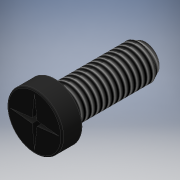
# Autodesk Inventor part: m5x12mmscrew
Saved by Autodesk Inventor 2018 (Build 220112000, 112)
## iProperties
Created: 2017-11-24
Part Number: m5x12mmscrew
Material: Generic
Document SubType Name: Modeling
Designer: g
Density: 1 g/cm^3
Appearance: Default
Author: g
Autodesk Inventor part; units mm, degrees
ref_plane "YZ Plane" through (0, 0, 0) normal (1, 0, 0) x (0, 1, 0)
ref_plane "XZ Plane" through (0, 0, 0) normal (0, 1, 0) x (-1, 0, 0)
ref_plane "XY Plane" through (0, 0, 0) normal (0, 0, 1) x (1, 0, 0)
sketch "Sketch1" plane through (0, 0, 0) normal (0, 1, 0) x (-1, 0, 0)
  circle A0 centre (0, 0) radius 2.5
  circle A1 centre (0, 0) radius 4
  dimension "d0" = 5
  dimension "d1" = 8
  constraints: 2 centre point, 2 coincident
  measures "d0" diameter of A0
  measures "d1" diameter of A1
extrude "Extrusion1" add sketch "Sketch1" along normal blind 15 contours A0
extrude "Extrusion2" add sketch "Sketch1" along normal blind 3
sketch "Sketch3" plane through (0, 0, 0) normal (0, -1, 0) x (1, 0, 0)
  line L0 (0, 0) -> (0, -0.4) construction
  circle A0 centre (0, 0) radius 4 projected
  line L1 (4, 0) -> (3.5, 0) construction
  line L2 (0, 0) -> (0, 0.4) construction
  line L3 (0.359, 0.359) -> (3.5, 0)
  line L4 (3.5, 0) -> (0.359, -0.359)
  line L5 (0.359, -0.359) -> (0, -3.5)
  line L6 (-0.359, -0.359) -> (0, -3.5)
  line L7 (-0.359, -0.359) -> (-3.5, 0)
  line L8 (-3.5, 0) -> (-0.359, 0.359)
  line L9 (-0.359, 0.359) -> (0, 3.5)
  line L10 (0, 3.5) -> (0.359, 0.359)
  dimension "d14" = 0.4
  dimension "d15" = 0.5
  dimension "d16" = 0.4
  dimension "d21" = 103.04
  dimension "d22" = 103.04
  dimension "d23" = 13.04
  dimension "d24" = 3.1615
  dimension "d25" = 3.1615
  constraints: 22 end point, 3 perpendicular, 2 horizontal, 2 vertical, 1 horizontal alignment, 1 other
  measures "d14" distance of L0.start L0.end
  measures "d15" distance of L1.start L1.end
  measures "d16" distance of L2.start L2.end
  measures "d21" angle of L8 L9
  measures "d22" angle of L3 L10
  measures "d23" angle of L10 L9
  measures "d24" distance of L8.end L9.end
  measures "d25" distance of L9.end L3.start
extrude "Extrusion3" cut sketch "Sketch3" against normal blind 2 contours L3 L4 L5 L6 L7 L8 L9 L10
fillet "Fillet1" radius 0.2 2 edges at (4, 0, 0) (4, 3, 0)
thread "Thread1" size "M5x0.8" class "6g" standard "ANSI Metric M Profile" full length
sketch "Sketch4" plane through (0, 15, 0) normal (0, 1, 0) x (1, 0, 0)
  circle A0 centre (0, 0) radius 2
  dimension "d31" = 4
  constraints: 1 centre point, 1 coincident
  measures "d31" diameter of A0
extrude "Extrusion4" add sketch "Sketch4" along normal blind 1
loft "Loft1" add section 1 edges at (-2, 16, 0) section 2 edges at (2.5, 15, 0)
thread "Thread2" size "R 5" standard "ISO Taper" full length
body "Solid1"
